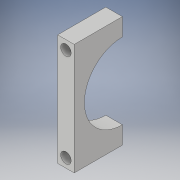
# Autodesk Inventor part: SujetadorColaVTOL
Saved by Autodesk Inventor 2019 (Build 230136000, 136)
## iProperties
Created: 2019-03-01
Part Number: SujetadorColaVTOL
Material: Generic
Document SubType Name: Modeling
Designer: Kenny
Density: 1 g/cm^3
Appearance: Default
Author: Kenny
Autodesk Inventor part; units mm, degrees
ref_plane "YZ Plane" through (0, 0, 0) normal (1, 0, 0) x (0, 1, 0)
ref_plane "XZ Plane" through (0, 0, 0) normal (0, 1, 0) x (-1, 0, 0)
ref_plane "XY Plane" through (0, 0, 0) normal (0, 0, 1) x (1, 0, 0)
sketch "Sketch1" plane through (0, 0, 0) normal (0, 0, 1) x (1, 0, 0)
  line L0 (0, 0) -> (5.5, 0)
  line L1 (5.5, 0) -> (5.5, 37)
  line L2 (5.5, 37) -> (0, 37)
  line L3 (0, 37) -> (0, 0)
  point P0 (2.75, 34)
  point P1 (2.75, 3)
  dimension "d7" = 5.5
  dimension "d8" = 37
  dimension "d9" = 31
  dimension "d10" = 3
  dimension "d11" = 2.75
  constraints: 8 end point, 2 parallel, 1 horizontal, 1 perpendicular, 1 vertical alignment
  measures "d7" distance of L2.end L1.end
  measures "d8" distance of L1.end L0.end
  measures "d9" distance of point (2.75, 3) point (2.75, 34)
  measures "d10" distance from line of L0 point (2.75, 3)
  measures "d11" distance from line of L1 point (2.75, 34)
extrude "Extrusion4" add sketch "Sketch1" along normal blind 16
sketch "Sketch6" plane through (0, 0, 0) normal (0, 0, 1) x (1, 0, 0)
  line L0 (0, 0) -> (5.5, 0)
  line L1 (5.5, 0) -> (5.5, 37)
  line L2 (5.5, 37) -> (0, 37)
  line L3 (0, 37) -> (0, 0)
  point P0 (2.75, 34)
  point P1 (2.75, 3)
  dimension "d45" = 5.5
  dimension "d46" = 37
  dimension "d47" = 31
  dimension "d48" = 3
  dimension "d49" = 2.75
  constraints: 8 end point, 2 parallel, 1 horizontal, 1 perpendicular, 1 vertical alignment
  measures "d45" distance of L2.end L1.end
  measures "d46" distance of L1.end L0.end
  measures "d47" distance of point (2.75, 3) point (2.75, 34)
  measures "d48" distance from line of L0 point (2.75, 3)
  measures "d49" distance from line of L1 point (2.75, 34)
hole "Hole3" at (2.75, 34, 0) at (2.75, 3, 0) direction (0, 0, 1) diameter 3.5 end through all
sketch "Sketch7" plane through (5.5, 0, 0) normal (1, 0, 0) x (0, 0, -1)
  line L0 (0, 0) -> (0, 37) projected
  arc A0 (0, 31.125) -> (0, 5.875) centre (0, 18.5) ccw
  line L1 (0, 31.125) -> (0, 5.875)
  dimension "d59" = 25.25
  constraints: 2 end point, 2 point on circle, 2 point on line, 1 centre point, 1 midpoint
  measures "d59" diameter of A0
extrude "Extrusion5" cut sketch "Sketch7" against normal blind 5.5
body "Solid3"
